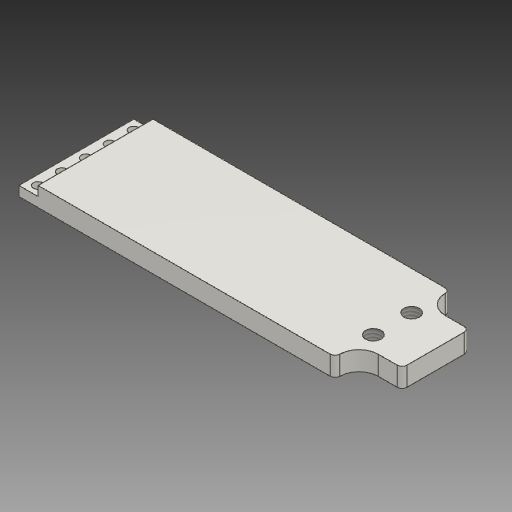
# Autodesk Inventor part: Kicker Eisen
Saved by Autodesk Inventor 2019.4 (Build 234330000, 330)
## iProperties
Part Number: Kicker Eisen
Material: Stahl, unlegiert
Document SubType Name: Modeling
Designer: rYan
Mass: 51.6105 g
Surface Area: 42.6729 cm^2
Volume: 6.57458 cm^3
Density: 7.85 g/cm^3
Appearance: Stahl
Author: rYan
Autodesk Inventor part; units mm, degrees
ref_plane "YZ Plane" through (0, 0, 0) normal (1, 0, 0) x (0, 1, 0)
ref_plane "XZ Plane" through (0, 0, 0) normal (0, 1, 0) x (-1, 0, 0)
ref_plane "XY Plane" through (0, 0, 0) normal (0, 0, 1) x (1, 0, 0)
sketch "Skizze1" plane through (0, 0, 0) normal (0, 0, 1) x (1, 0, 0)
  line L0 (0, 12) -> (66, 12)
  line L1 (66, -12) -> (0, -12)
  line L2 (0, -12) -> (0, 12)
  line L3 (-15, 0) -> (90, 0) projected
  line L4 (66, -7) -> (75, -7)
  line L5 (75, -7) -> (75, 7)
  line L6 (75, 7) -> (66, 7)
  line L7 (66, 12) -> (66, 7)
  line L8 (66, -7) -> (66, -12)
  point P0 (0, 0)
  dimension "d0" = 24
  dimension "d1" = 66
  dimension "d29" = 14
  dimension "d30" = 9
  constraints: 16 end point, 4 parallel, 3 perpendicular, 2 horizontal, 1 collinear, 1 midpoint, 2 other
  measures "d0" distance of L1.end L0.start
  measures "d1" distance of L0.start L0.end
  measures "d29" distance of L4.end L5.end
  measures "d30" distance of L5.end L6.end
extrude "Extrusion1" add sketch "Skizze1" along normal blind 4
sketch "Skizze2" plane through (0, 0, 4) normal (0, 0, 1) x (1, 0, 0)
  line L0 (66, 12) -> (0, 12) projected
  line L1 (0, 12) -> (0, -12) projected
  line L2 (0, 12) -> (4, 12)
  line L3 (4, 12) -> (4, -12)
  line L4 (4, -12) -> (0, -12)
  line L5 (0, -12) -> (0, 12)
  point P0 (0, 0)
  dimension "d4" = 4
  constraints: 8 end point, 2 parallel, 1 horizontal, 1 perpendicular, 1 point on line
  measures "d4" distance between parallel lines of L1 L3
extrude "Extrusion2" cut sketch "Skizze2" against normal blind 2
sketch "Skizze3" plane through (0, 0, 2) normal (0, 0, 1) x (1, 0, 0)
  line L0 (0, 16.8) -> (0, -16.8) projected
  line L1 (-15, 0) -> (90, 0) projected
  point P0 (0, 0)
  point P1 (2, 0)
  dimension "d7" = 2
  constraints: 1 point on line
  measures "d7" distance from line of L0 point (2, 0)
hole "Bohrung1" at (2, 0, 2) direction (0, 0, -1) diameter 2 end through all
pattern_linear "Rechteckige Anordnung1" count 5 spacing 5 along (0, 1, 0) of "Bohrung1" first direction both ways yes
sketch "Skizze4" plane through (0, 0, 4) normal (0, 0, 1) x (1, 0, 0)
  line L0 (-15, 0) -> (90, 0) projected
  line L1 (66, -12) -> (66, 12) projected
  line L2 (75, -7) -> (75, 7) construction
  point P0 (0, 0)
  point P1 (66, 4)
  point P2 (66, -4)
  dimension "d31" = 8
  dimension "d36" = 0
  constraints: 1 symmetric about line
  measures "d31" distance of point (66, -4) point (66, 4)
  measures "d36" distance from line of point (66, -4) L1
hole "Bohrung2" at (66, -4, 4) at (66, 4, 4) direction (0, 0, -1) diameter 3.242 end through all thread size "M4x0.7" class "6H" standard "ISO Metric profile"
fillet "Rundung1" radius 4 2 edges at (66, -7, 2) (66, 7, 2)
fillet "Rundung2" radius 1 4 edges at (66, -12, 2) (66, 12, 2) (75, -7, 2) (75, 7, 2)
